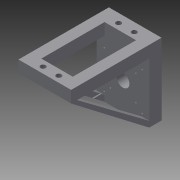
# Autodesk Inventor part: Part1
Saved by Autodesk Inventor 2015 (Build 190159000, 159)
## iProperties
Created: 2015-03-24
Part Number: Part1
Material: Generic
Document SubType Name: Modeling
Designer: nelsona
Density: 1 g/cm^3
Appearance: Default
Author: nelsona
Autodesk Inventor part; units mm, degrees
ref_plane "YZ Plane" through (0, 0, 0) normal (1, 0, 0) x (0, 1, 0)
ref_plane "XZ Plane" through (0, 0, 0) normal (0, 1, 0) x (-1, 0, 0)
ref_plane "XY Plane" through (0, 0, 0) normal (0, 0, 1) x (1, 0, 0)
sketch "Sketch1" plane through (0, 0, 0) normal (0, 1, 0) x (-1, 0, 0)
  line L0 (0, 0) -> (-20.3922, 0)
  line L1 (-20.3922, 0) -> (-20.3922, -40.9956)
  line L2 (-20.3922, -40.9956) -> (0, -40.9956)
  line L3 (0, -40.9956) -> (0, 0)
  line L4 (1.8083, 7.7679) -> (6.8846, 7.9604)
  line L5 (-22.5838, -48.6642) -> (-27.2554, -50.6597)
  line L6 (6.8846, 7.9604) -> (-27.2554, 7.9604)
  line L7 (-27.2554, 7.9604) -> (-27.2554, -50.6597)
  line L8 (-27.2554, -50.6597) -> (6.8846, -50.6597)
  line L9 (6.8846, -50.6597) -> (6.8846, 7.9604)
  circle A0 centre (-5.0927, 3.9878) radius 1.651
  circle A1 centre (-15.2781, 3.9878) radius 1.651
  circle A2 centre (-5.0927, -44.9834) radius 1.651
  circle A3 centre (-15.2781, -44.9834) radius 1.651
  dimension "d0" = 40.9956
  dimension "d2" = 7.9756
  dimension "d3" = 5.08
  dimension "d4" = 7.9756
  dimension "d5" = 5.08
  dimension "d6" = 3.302
  dimension "d7" = 3.302
  dimension "d8" = 3.302
  dimension "d9" = 3.302
  dimension "d24" = 6.8846
  dimension "d25" = 6.8633
  constraints: 20 end point, 4 centre point, 4 parallel, 2 horizontal, 2 perpendicular
  measures "d0" distance of L1.end L0.end
  measures "d2" distance of L0.start L4.start
  measures "d3" distance of L4.start L4.end
  measures "d4" distance of L1.end L5.start
  measures "d5" distance of L5.start L5.end
  measures "d6" diameter of A0
  measures "d7" diameter of A1
  measures "d8" diameter of A2
  measures "d9" diameter of A3
  measures "d24" distance between parallel lines of L9 L3
  measures "d25" distance between parallel lines of L7 L1
extrude "Extrusion1" add sketch "Sketch1" along normal blind 7.62
sketch "Sketch2" plane through (0, 0, 0) normal (0, -1, 0) x (1, 0, 0)
  line L0 (27.2554, 7.9604) -> (27.2554, -50.6597) projected
  line L1 (27.2554, -42.6841) -> (-6.8846, -42.6841)
  line L2 (-6.8846, -42.6841) -> (-6.8846, -50.6597)
  line L3 (-6.8846, -50.6597) -> (27.2554, -50.6597)
  line L4 (27.2554, -50.6597) -> (27.2554, -42.6841)
  point P0 (0, 0)
  constraints: 8 end point, 2 parallel, 1 horizontal, 1 perpendicular, 1 point on line
extrude "Extrusion2" add sketch "Sketch2" along normal blind 38.862
sketch "Sketch3" plane through (27.2554, 0, 7.9604) normal (1, 0, 0) x (0, 0, -1)
  line L0 (0, 0) -> (50.6445, -38.862)
  line L1 (50.6445, -38.862) -> (50.6445, -35.052)
  line L2 (50.6445, 0) -> (50.6445, -38.862) projected
  line L3 (0, 0) -> (3.81, 0)
  line L4 (0, 0) -> (50.6445, 0) projected
  line L5 (3.81, 0) -> (50.6445, -35.052)
  point P0 (7.9604, 0)
  dimension "d14" = 3.81
  dimension "d15" = 3.81
  constraints: 8 end point, 2 point on line
  measures "d14" distance of L0.end L1.end
  measures "d15" distance of L0.start L3.end
extrude "Extrusion3" add sketch "Sketch3" against normal blind 5.08 contours L3 L5 L1 L0
sketch "Sketch4" plane through (-6.8846, 0, -42.6841) normal (-1, 0, 0) x (0, 0, 1)
  line L0 (0, -38.862) -> (0, -35.052)
  line L1 (0, 0) -> (0, -38.862) projected
  line L2 (48.9049, 0) -> (45.0949, 0)
  line L3 (0, 0) -> (50.6445, 0) projected
  line L4 (45.0949, 0) -> (0, -35.052)
  line L5 (0, -38.862) -> (50.6445, 0)
  line L6 (50.6445, 0) -> (45.0949, 0)
  point P0 (42.6841, 0)
  dimension "d18" = 3.81
  dimension "d19" = 3.81
  constraints: 10 end point, 2 point on line
  measures "d18" distance of L0.start L0.end
  measures "d19" distance of L2.start L2.end
extrude "Extrusion4" add sketch "Sketch4" against normal blind 5.08 contours L0 L4 L2 L3 L5
sketch "Sketch5" plane through (27.2554, 7.62, -50.6597) normal (0, 0, -1) x (-1, 0, 0)
  line L0 (2.6344, -13.9998) -> (31.438, -13.9998)
  line L1 (31.438, -13.9998) -> (31.438, -42.8034)
  line L2 (31.438, -42.8034) -> (2.6344, -42.8034)
  line L3 (2.6344, -42.8034) -> (2.6344, -13.9998)
  line L4 (31.438, -13.9998) -> (2.6344, -42.8034)
  line L5 (2.6344, -13.9998) -> (31.438, -42.8034)
  line L6 (17.0362, -28.4016) -> (25.2981, -20.1398)
  line L7 (17.0362, -28.4016) -> (8.7744, -20.1398)
  line L8 (17.0362, -28.4016) -> (8.7744, -36.6634)
  line L9 (17.0362, -28.4016) -> (25.2981, -36.6634)
  line L10 (17.0362, -28.4016) -> (29.3572, -16.0807)
  line L11 (17.0362, -28.4016) -> (4.7153, -16.0807)
  line L12 (17.0362, -28.4016) -> (4.7153, -40.7225)
  line L13 (17.0362, -28.4016) -> (29.3572, -40.7225)
  circle A0 centre (25.2981, -20.1398) radius 0.508
  circle A1 centre (29.3572, -16.0807) radius 0.508
  circle A2 centre (4.7153, -16.0807) radius 0.508
  circle A3 centre (8.7744, -20.1398) radius 0.508
  circle A4 centre (8.7744, -36.6634) radius 0.508
  circle A5 centre (4.7153, -40.7225) radius 0.508
  line L14 (17.0362, -28.4016) -> (25.2981, -36.6634)
  circle A6 centre (25.2981, -36.6634) radius 0.508
  circle A7 centre (29.3572, -40.7225) radius 0.508
  circle A8 centre (17.0362, -28.4016) radius 4.1783
  point P0 (27.2554, -7.62)
  dimension "d22" = 28.8036
  dimension "d26" = 28.8036
  dimension "d27" = 11.684
  dimension "d28" = 11.684
  dimension "d29" = 11.684
  dimension "d30" = 17.4244
  dimension "d31" = 17.4244
  dimension "d32" = 17.4244
  dimension "d33" = 17.4244
  dimension "d34" = 1.016
  dimension "d35" = 1.016
  dimension "d36" = 1.016
  dimension "d37" = 1.016
  dimension "d38" = 1.016
  dimension "d39" = 1.016
  dimension "d40" = 11.684
  dimension "d41" = 1.016
  dimension "d42" = 1.016
  dimension "d43" = 8.3566
  constraints: 30 end point, 9 centre point, 9 coincident, 8 point on line, 2 parallel, 1 collinear, 1 horizontal, 1 midpoint, 1 perpendicular
  measures "d22" distance of L1.end L2.end
  measures "d26" distance of L0.end L1.end
  measures "d27" distance of L6.start L6.end
  measures "d28" distance of L6.start L7.end
  measures "d29" distance of L6.start L8.end
  measures "d30" distance of L6.start L10.end
  measures "d31" distance of L6.start L11.end
  measures "d32" distance of L6.start L12.end
  measures "d33" distance of L6.start L13.end
  measures "d34" diameter of A0
  measures "d35" diameter of A1
  measures "d36" diameter of A2
  measures "d37" diameter of A3
  measures "d38" diameter of A4
  measures "d39" diameter of A5
  measures "d40" distance of L6.start L9.end
  measures "d41" diameter of A6
  measures "d42" diameter of A7
  measures "d43" diameter of A8
extrude "Extrusion5" cut sketch "Sketch5" against normal through all contours A2 L5 | L5 A2 | A1 L4 | L4 A1 | A5 L4 | L4 A5 | A7 L5 | L5 A7 | A3 L5 | L5 A3 | A0 L4 | L4 A0 | A4 L4 | L4 A4 | A6 L5 | L5 A6 | A8 L4 L5 | L5 L4 A8 | A8 L5 L4 | L4 L5 A8
body "Solid1"
